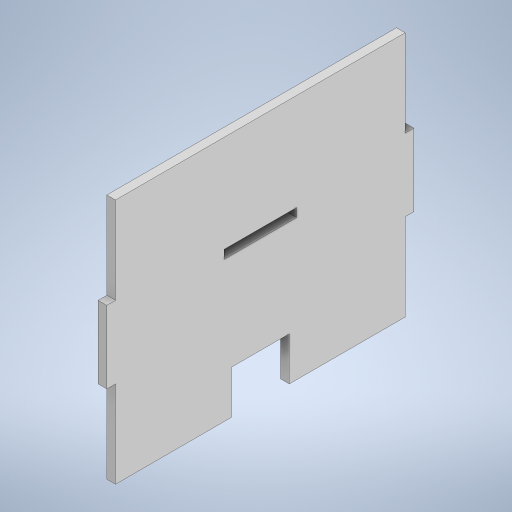
# Autodesk Inventor part: Depan
Saved by Autodesk Inventor 2023 (Build 270158000, 158)
## iProperties
Created: 2023-02-07
Part Number: Depan
Material: Generic
Document SubType Name: Modeling
Designer: Asus
Density: 1 g/cm^3
Appearance: Default
Author: Asus
Autodesk Inventor part; units mm, degrees
ref_plane "YZ Plane" through (0, 0, 0) normal (1, 0, 0) x (0, 1, 0)
ref_plane "XZ Plane" through (0, 0, 0) normal (0, 1, 0) x (-1, 0, 0)
ref_plane "XY Plane" through (0, 0, 0) normal (0, 0, 1) x (1, 0, 0)
sketch "Sketch1" plane through (0, 0, 0) normal (1, 0, 0) x (0, 1, 0)
  line L0 (0, -100) -> (30, -100)
  line L1 (30, -100) -> (30, -103)
  line L2 (30, -103) -> (55, -103)
  line L3 (55, -103) -> (55, -100)
  line L4 (55, -100) -> (85, -100)
  line L5 (85, -100) -> (85, 0)
  line L6 (85, 0) -> (55, 0)
  line L7 (55, 0) -> (55, 3)
  line L8 (55, 3) -> (30, 3)
  line L9 (30, 3) -> (30, 0)
  line L10 (30, 0) -> (0, 0)
  line L11 (0, 0) -> (0, -40)
  line L12 (0, -40) -> (15, -40)
  line L13 (15, -40) -> (15, -60)
  line L14 (15, -60) -> (0, -60)
  line L15 (0, -60) -> (0, -100)
  line L16 (0, -50) -> (52.5, -50) construction
  line L17 (52.5, -50) -> (80, -50) construction
  line L18 (0, -50) -> (48.5, -50) construction
  line L19 (48.5, -50) -> (51.5, -50) construction
  line L20 (48.5, -50) -> (48.5, -62.5)
  line L21 (48.5, -62.5) -> (51.5, -62.5)
  line L22 (51.5, -62.5) -> (51.5, -37.5)
  line L23 (51.5, -37.5) -> (48.5, -37.5)
  line L24 (48.5, -37.5) -> (48.5, -50)
  dimension "d0" = 100
  dimension "d1" = 30
  dimension "d2" = 3
  dimension "d3" = 25
  dimension "d5" = 30
  dimension "d6" = 100
  dimension "d7" = 30
  dimension "d8" = 3
  dimension "d9" = 25
  dimension "d10" = 3
  dimension "d11" = 30
  dimension "d15" = 15
  dimension "d16" = 20
  dimension "d23" = 27.5
  dimension "d25" = 48.5
  dimension "d26" = 3
  dimension "d27" = 12.5
  dimension "d28" = 3
  dimension "d29" = 25
  dimension "d30" = 3
  dimension "d31" = 12.5
  constraints: 50 end point, 10 perpendicular, 10 point on line, 2 horizontal, 2 vertical
  measures "d0" distance of L10.end L0.start
  measures "d1" distance of L0.start L0.end
  measures "d2" distance of L0.end L1.end
  measures "d3" distance of L1.end L2.end
  measures "d5" distance of L3.end L4.end
  measures "d6" distance of L4.end L5.end
  measures "d7" distance of L5.end L6.end
  measures "d8" distance of L6.end L7.end
  measures "d9" distance of L7.end L8.end
  measures "d10" distance of L8.end L9.end
  measures "d11" distance of L9.end L10.end
  measures "d15" distance of L11.end L12.end
  measures "d16" distance of L12.end L13.end
  measures "d23" distance of L16.end L17.end
  measures "d25" distance of L16.start L18.end
  measures "d26" distance of L18.end L19.end
  measures "d27" distance of L18.end L20.end
  measures "d28" distance of L20.end L21.end
  measures "d29" distance of L21.end L22.end
  measures "d30" distance of L22.end L23.end
  measures "d31" distance of L23.end L18.end
extrude "Extrusion2" add sketch "Sketch1" along normal blind 3
body "Solid2"
